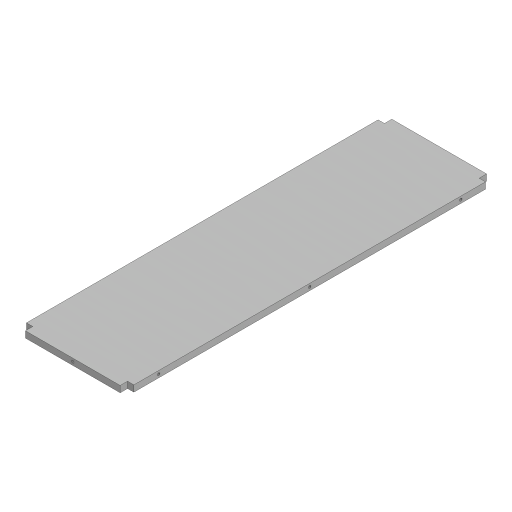
# Autodesk Inventor part: I Bodenplatte
Saved by Autodesk Inventor 2023 (Build 270158000, 158)
## iProperties
Created: 2022-09-18
Part Number: I Bodenplatte
Material: PVC, hart
Document SubType Name: Modeling
Designer: musati
Density: 1.29 g/cm^3
Appearance: Light Gray
Author: musati
Autodesk Inventor part; units mm, degrees
ref_plane "YZ Plane" through (0, 0, 0) normal (1, 0, 0) x (0, 1, 0)
ref_plane "XZ Plane" through (0, 0, 0) normal (0, 1, 0) x (-1, 0, 0)
ref_plane "XY Plane" through (0, 0, 0) normal (0, 0, 1) x (1, 0, 0)
sketch "Skizze1" plane through (0, 0, 0) normal (0, 0, 1) x (1, 0, 0)
  line L0 (-71.4, 0) -> (71.4, 0) projected
  line L1 (0, -4.2) -> (0, 4.2) projected
  line L2 (-51, -3) -> (51, -3)
  line L3 (51, -3) -> (51, 3)
  line L4 (51, 3) -> (-51, 3)
  line L5 (-51, 3) -> (-51, -3)
  line L6 (-51, -3) -> (51, 3) construction
  line L7 (51, -3) -> (-51, 3) construction
  point P0 (0, 0)
  dimension "d0" = 102
  dimension "d1" = 6
  constraints: 12 end point, 2 midpoint, 2 parallel, 1 horizontal, 1 perpendicular
  measures "d0" distance of L4.end L3.end
  measures "d1" distance of L3.end L2.end
extrude "Extrusion1" add sketch "Skizze1" against normal blind 348
sketch "Skizze2" plane through (-51, 3, 0) normal (0, 1, 0) x (1, 0, 0)
  line L0 (102, 0) -> (0, 0) projected
  line L1 (102, 0) -> (102, 348) projected
  line L2 (0, 348) -> (102, 348) projected
  line L3 (0, 0) -> (0, 348) projected
  line L4 (-20.4, 0) -> (122.4, 0) projected
  line L5 (51, 417.6) -> (51, -69.6) projected
  line L6 (0, 0) -> (102, 0) projected
  line L7 (0, 0) -> (6, 0)
  line L8 (6, 0) -> (6, 7)
  line L9 (6, 7) -> (0, 7)
  line L10 (0, 7) -> (0, 0)
  line L11 (102, 0) -> (96, 0)
  line L12 (96, 0) -> (96, 7)
  line L13 (96, 7) -> (102, 7)
  line L14 (102, 7) -> (102, 0)
  line L15 (102, 0) -> (102, 348) projected
  line L16 (102, 348) -> (96, 348)
  line L17 (96, 348) -> (96, 341)
  line L18 (96, 341) -> (102, 341)
  line L19 (102, 341) -> (102, 348)
  line L20 (102, 348) -> (0, 348) projected
  line L21 (0, 348) -> (6, 348)
  line L22 (6, 348) -> (6, 341)
  line L23 (6, 341) -> (0, 341)
  line L24 (0, 341) -> (0, 348)
  point P0 (51, 0)
  point P1 (0, 7)
  point P2 (6, 0)
  dimension "d4" = 6
  dimension "d5" = 7
  dimension "d6" = 6
  dimension "d7" = 7
  dimension "d8" = 6
  constraints: 32 end point, 8 parallel, 4 horizontal, 4 perpendicular, 3 point on line
  measures "d4" distance of L9.end L8.end
  measures "d5" distance of L8.end L7.end
  measures "d6" distance of L12.end L13.end
  measures "d7" distance of L17.end L16.end
  measures "d8" distance of L17.end L18.end
extrude "Extrusion2" cut sketch "Skizze2" against normal blind 348 contours L0 L12 L13 L1 | L18 L17 L2 L1 | L0 L3 L9 L8 | L22 L23 L3 L2
sketch "Skizze3" plane through (51, 3, -7) normal (1, 0, 0) x (0, 0, -1)
  line L0 (334, -6) -> (334, 0) projected
  line L1 (0, 0) -> (334, 0) projected
  line L2 (0, 0) -> (0, -6) projected
  line L3 (0, -6) -> (334, -6) projected
  point P0 (-7, -3)
  point P1 (23.5, -3)
  point P2 (167, -3)
  point P3 (310.5, -3)
  dimension "d11" = 23.5
  dimension "d12" = 23.5
  dimension "d13" = 167
  measures "d11" distance from line of point (23.5, -3) L2
  measures "d12" distance from line of point (310.5, -3) L0
  measures "d13" distance from line of point (167, -3) L2
hole "Bohrung1" at (51, 0, -30.5) at (51, 0, -174) at (51, 0, -317.5) direction (-1, 0, 0) diameter 2.459 depth 8.8 tip angle 118 thread size "M3x0.5" class "6H" standard "ANSI Metric M Profile"
sketch "Skizze4" plane through (0, 0, 0) normal (0, 0, 1) x (1, 0, 0)
  line L0 (-45, 3) -> (-45, -3) projected
  line L1 (-45, -3) -> (45, -3) projected
  line L2 (45, -3) -> (45, 3) projected
  line L3 (45, 3) -> (-45, 3) projected
  line L4 (-71.4, 0) -> (71.4, 0) projected
  line L5 (0, -4.2) -> (0, 4.2) projected
  point P0 (0, 0)
  point P1 (0, 0)
  constraints: 1 coincident
hole "Bohrung2" at (0, 0, 0) direction (0, 0, -1) diameter 2.459 depth 17 tip angle 118 thread size "M3x0.5" class "6H" standard "ANSI Metric M Profile"
sketch "Skizze5" plane through (-51, 3, -341) normal (-1, 0, 0) x (0, 0, 1)
  line L0 (334, -6) -> (334, 0) projected
  line L1 (334, 0) -> (0, 0) projected
  line L2 (0, 0) -> (0, -6) projected
  line L3 (334, -6) -> (0, -6) projected
  circle A0 centre (310.5, -3) radius 1.2295 projected
  circle A1 centre (167, -3) radius 1.2295 projected
  circle A2 centre (23.5, -3) radius 1.2295 projected
  line L4 (341, -7.2) -> (341, 1.2) projected
  line L5 (-76.6, -3) -> (410.6, -3) projected
  circle A3 centre (23.5, -3) radius 1.2295 projected
  point P0 (341, -3)
  constraints: 3 coincident
hole "Bohrung3" at (-51, 0, -317.5) at (-51, 0, -174) at (-51, 0, -30.5) direction (1, 0, 0) diameter 2.459 depth 17 tip angle 118 thread size "M3x0.5" class "6H" standard "ANSI Metric M Profile"
